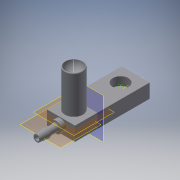
# Autodesk Inventor part: 9mm_holder_JL_rev_6
Saved by Autodesk Inventor 2019 (Build 230136000, 136)
## iProperties
Created: 2008-05-07
Part Number: 9mm_holder_JL_rev_6
Document SubType Name: Modeling
Designer: osbornej
Density: 1 g/cm^3
Mass: 5.78507 g
Surface Area: 32.2527 cm^2
Volume: 5.78507 cm^3
Material: Generic
Appearance: Default
Author: osbornej
Autodesk Inventor part; units mm, degrees
ref_plane "YZ Plane" through (0, 0, 0) normal (1, 0, 0) x (0, 1, 0)
ref_plane "XZ Plane" through (0, 0, 0) normal (0, 1, 0) x (-1, 0, 0)
ref_plane "XY Plane" through (0, 0, 0) normal (0, 0, 1) x (1, 0, 0)
sketch "Sketch1" plane through (0, 0, 0) normal (0, 0, 1) x (1, 0, 0)
  line L0 (6.5833, -5.9802) -> (1.6807, -5.9802)
  line L1 (1.6807, -5.9802) -> (1.6807, 22.1437)
  line L2 (1.6807, 22.1437) -> (2.1004, 22.1437)
  line L3 (6.5833, 18.0359) -> (6.5833, -5.9802)
  arc A0 (2.1004, 22.1437) -> (6.5833, 18.0359) centre (6.5833, 22.5359) ccw
  line L4 (6.5833, 22.5359) -> (2.1004, 22.1437) construction
  line L5 (6.5833, 22.5359) -> (6.5833, 18.0359) construction
  dimension "d136" = 4.5
  dimension "d137" = 85
  constraints: 13 end point, 2 perpendicular, 2 point on circle, 1 centre point, 1 parallel, 1 vertical
  measures "d136" radius of A0
  measures "d137" angle of L4 L5
revolve "Revolution1" add sketch "Sketch1" angle 360 about axis through (6.5833, 18.0359, 0) along (0, -1, 0)
sketch "Sketch4" plane through (6.5833, -5.9802, 0) normal (0, -1, 0) x (1, 0, 0)
  line L0 (7.9168, 7.2925) -> (-7.3232, 7.2925)
  line L1 (-7.3232, 7.2925) -> (-7.3232, -33.3475)
  line L2 (-7.3232, -33.3475) -> (7.9168, -33.3475)
  line L3 (7.9168, -33.3475) -> (7.9168, 7.2925)
  circle A0 centre (0, 0) radius 4.9026
  point P0 (-6.5833, 0)
  point P1 (12.6896, -12.6896)
  point P2 (12.6896, 12.6896)
  point P3 (-12.6896, 12.6896)
  point P4 (-12.6896, -12.6896)
  dimension "d115" = 15.24
  dimension "d116" = 40.64
  constraints: 8 end point, 1 centre point, 1 horizontal, 1 parallel, 1 perpendicular
  measures "d115" distance of L2.end L1.end
  measures "d116" distance of L0.end L1.end
ref_plane "Work Plane3" through (6.5833, 0.3698, 0) normal (0, 1, 0) x (1, 0, 0)
sketch "Sketch8" plane through (6.5833, 0.3698, 0) normal (0, 1, 0) x (1, 0, 0)
  point P0 (-6.5833, 0)
  point P1 (0.0035, 25.4064)
extrude "Extrusion4" add sketch "Sketch4" against normal blind 7.62
sketch "Sketch10" plane through (6.5833, 0.3698, 0) normal (0, 1, 0) x (1, 0, 0)
  point P0 (-6.5833, 0)
  point P1 (0, 0)
hole "Hole12" at (6.5833, 0.3698, 0) direction (0, 1, 0) diameter 1.27 end through all
sketch "Sketch11" plane through (6.5833, 0.3698, 0) normal (0, 1, 0) x (1, 0, 0)
  circle A0 centre (0, 0) radius 4.9026 projected
  point P0 (-6.5833, 0)
  point P1 (0, 4.9026)
  constraints: 1 vertical alignment, 1 other
ref_plane "Work Plane5" through (6.5833, 0.3698, -4.9026) normal (0, 0, -1) x (-1, 0, 0)
hole "Hole14" at (6.5833, 0.3698, 0) direction (0, 1, 0) diameter 5.08 depth 10.16 tip angle 118
sketch "Sketch13" plane through (-0.7399, -5.9802, 7.2925) normal (0, -1, 0) x (1, 0, 0)
  circle A0 centre (7.3232, -7.2925) radius 4.191
  point P0 (0.7399, -7.2925)
  dimension "d168" = 8.382
  constraints: 1 centre point, 1 coincident
  measures "d168" diameter of A0
extrude "Extrusion5" [suppressed]
fillet "Fillet1" radius 0.508 1 edges at (11.4859, 22.1437, 0)
fillet "Fillet2" radius 0.1016 1 edges at (11.0655, 22.1361, 0)
sketch "Sketch15" plane through (6.5833, 1.6398, 0) normal (0, 1, 0) x (1, 0, 0)
  circle A0 centre (0, 0) radius 2.54
  point P0 (-6.5833, 0)
  constraints: 1 centre point
extrude "Extrusion6" cut sketch "Sketch15" against normal blind 6.35
sketch "Sketch16" plane through (-0.7399, -5.9802, 7.2925) normal (0, 0, 1) x (1, 0, 0)
  circle A0 centre (7.3391, 4.1422) radius 1.9019
  point P0 (0.7399, 5.9802)
  constraints: 1 centre point
extrude "Extrusion7" cut sketch "Sketch16" against normal blind 6.35
ref_plane "Work Plane6" through (6.5992, -1.838, 7.2925) normal (0, 1, 0) x (-1, 0, 0)
sketch "Sketch17" plane through (6.5992, -1.838, 7.2925) normal (0, 1, 0) x (-1, 0, 0)
  line L0 (7.3391, 0) -> (-7.9009, 0) projected
  line L1 (3.0545, 0) -> (3.0545, 2.4437)
  line L2 (3.0545, 2.4437) -> (2.3921, 2.4437)
  line L3 (0, 0) -> (0, 3.2191)
  line L4 (1.15, 0) -> (1.15, 12.7089)
  arc A0 (1.88, 2.7813) -> (2.3921, 2.4437) centre (2.3921, 3.0009) ccw
  line L5 (1.88, 2.7813) -> (1.88, 7.7813)
  line L6 (1.88, 7.7813) -> (2.413, 7.7813)
  line L7 (0, 23.6283) -> (0, -51.3514) projected
  line L8 (1.88, 7.7813) -> (1.88, 12.8613) construction
  line L9 (2.413, 7.7813) -> (1.8805, 12.7575)
  arc A1 (1.8805, 12.7575) -> (1.7428, 12.8813) centre (1.7428, 12.7427) ccw
  arc A2 (1.3224, 12.8813) -> (1.15, 12.7089) centre (1.3224, 12.7089) ccw
  line L10 (1.3224, 12.8813) -> (1.7428, 12.8813)
  point P0 (6.5992, -7.2925)
  dimension "d187" = 1.15
  dimension "d188" = 5
  dimension "d189" = 2.413
  dimension "d190" = 1.88
  dimension "d191" = 5.08
  constraints: 18 end point, 6 point on circle, 5 tangent, 4 vertical, 3 centre point, 3 horizontal, 3 point on line, 2 coincident, 1 collinear, 1 perpendicular
  measures "d187" distance between parallel lines of L3 L4
  measures "d188" distance of L5.start L5.end
  measures "d189" distance from line of L6.end L7
  measures "d190" distance between parallel lines of L5 L3
  measures "d191" distance of L5.end L8.end
revolve "Revolution2" add sketch "Sketch17" angle 360 about axis through (6.5992, -1.838, 7.2925) along (0, 0, -1)
sketch "Sketch18" plane through (6.5833, 1.6398, 0) normal (0, 1, 0) x (1, 0, 0)
  circle A0 centre (0, 0) radius 0.635 projected
  point P0 (-6.5833, 0)
  point P1 (0, 25.4)
  dimension "d197" = 25.4
  constraints: 1 coincident
  measures "d197" distance of A0.centre point (0, 25.4)
hole "Hole16" at (6.5833, 1.6398, -25.4) direction (0, -1, 0) diameter 4.4958 end through all counterbore diameter 8.4328 counterbore depth 4.572 clearance for "Flat Head Machine Screw (82)" size "#8" standard "Ansi Unified Screw Threads"
body "Solid1"
